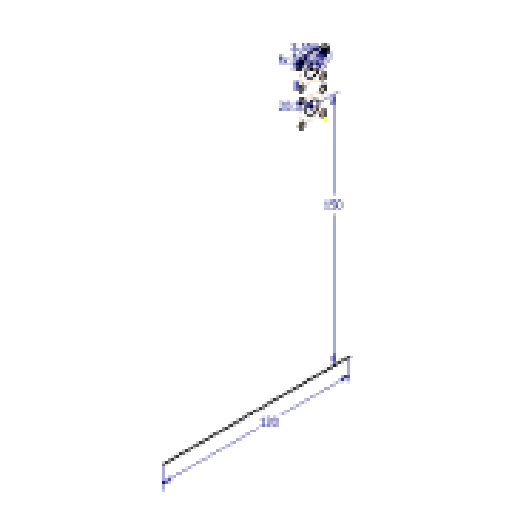
# Autodesk Inventor part: PlatformSidePlate
Saved by Autodesk Inventor 2023 (Build 270158000, 158)
## iProperties
Created: 2022-11-09
Part Number: PlatformSidePlate
Material: Polycarbonate, Smoke
Document SubType Name: Modeling
Designer: deli
Density: 1.2 g/cm^3
Appearance: Polycarbonate - Smoked
Author: deli
Autodesk Inventor part; units mm, degrees
ref_plane "YZ Plane" through (0, 0, 0) normal (1, 0, 0) x (0, 1, 0)
ref_plane "XZ Plane" through (0, 0, 0) normal (0, 1, 0) x (-1, 0, 0)
ref_plane "XY Plane" through (0, 0, 0) normal (0, 0, 1) x (1, 0, 0)
sketch "Sketch1" plane through (0, 0, 0) normal (1, 0, 0) x (0, 1, 0)
  circle A0 centre (11.9223, 3.3524) radius 4
  circle A1 centre (-8.6517, 3.3524) radius 4
  circle A2 centre (18.8371, 10.2672) radius 1.778
  circle A3 centre (18.8371, -3.5624) radius 1.778
  circle A4 centre (5.0075, 10.2672) radius 1.778
  circle A5 centre (5.0075, -3.5624) radius 1.778
  circle A6 centre (-1.7369, 10.2672) radius 1.778
  circle A7 centre (-1.7369, -3.5624) radius 1.778
  circle A8 centre (-15.5665, 10.2672) radius 1.778
  circle A9 centre (-15.5665, -3.5624) radius 1.778
  line L0 (18.8371, 10.2672) -> (18.8371, -3.5624) construction
  line L1 (18.8371, -3.5624) -> (5.0075, -3.5624) construction
  line L2 (5.0075, -3.5624) -> (5.0075, 10.2672) construction
  line L3 (5.0075, 10.2672) -> (18.8371, 10.2672) construction
  line L4 (-1.7369, 10.2672) -> (-1.7369, -3.5624) construction
  line L5 (-1.7369, -3.5624) -> (-15.5665, -3.5624) construction
  line L6 (-15.5665, -3.5624) -> (-15.5665, 10.2672) construction
  line L7 (-15.5665, 10.2672) -> (-1.7369, 10.2672) construction
  line L8 (18.8371, 10.2672) -> (5.0075, -3.5624) construction
  line L9 (-1.7369, 10.2672) -> (-15.5665, -3.5624) construction
  line L10 (-27.7907, 133.0654) -> (-27.7907, -6.9346)
  arc A10 (18.8371, -6.9346) -> (22.2093, -3.5624) centre (18.8371, -3.5624) ccw
  line L11 (22.2093, 133.0654) -> (22.2093, -3.5624)
  line L12 (-27.7907, 133.0654) -> (22.2093, 133.0654)
  line L13 (-27.7907, -6.9346) -> (18.8371, -6.9346)
  point P0 (0, 0)
  dimension "d0" = 8
  dimension "d1" = 3.556
  dimension "d2" = 19.558
  dimension "d3" = 20.574
  dimension "d5" = 13.8296
  dimension "d6" = 140
  dimension "d11" = 39.713
  constraints: 28 end point, 11 centre point, 8 equal radius, 7 perpendicular, 3 coincident, 3 equal length, 2 horizontal, 2 midpoint, 2 point on circle, 2 vertical, 1 collinear, 1 parallel, 1 tangent
  measures "d0" diameter of A0
  measures "d1" diameter of A2
  measures "d2" distance of L0.start L1.end
  measures "d3" distance of A1.centre A0.centre
  measures "d5" distance of L0.start L0.end
  measures "d6" distance of L10.start L10.end
  measures "d11" distance from line of A0.centre L10
extrude "Extrusion1" add sketch "Sketch1" along normal blind 3.175
body "Solid1"
